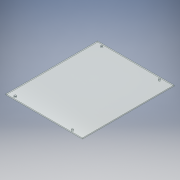
# Autodesk Inventor part: Perspex base
Saved by Autodesk Inventor 2019 (Build 230136000, 136)
## iProperties
Created: 2021-03-22
Part Number: Perspex base
Material: Glass
Document SubType Name: Modeling
Designer: User
Density: 2.18 g/cm^3
Appearance: Clear
Author: User
Autodesk Inventor part; units mm, degrees
ref_plane "YZ Plane" through (0, 0, 0) normal (1, 0, 0) x (0, 1, 0)
ref_plane "XZ Plane" through (0, 0, 0) normal (0, 1, 0) x (-1, 0, 0)
ref_plane "XY Plane" through (0, 0, 0) normal (0, 0, 1) x (1, 0, 0)
sketch "Sketch1" plane through (0, 0, 0) normal (0, 1, 0) x (-1, 0, 0)
  line L0 (300, 0) -> (-11, 0)
  line L1 (-11, 0) -> (-11, -373)
  line L2 (-11, -373) -> (300, -373)
  line L3 (300, -373) -> (300, 0)
  point P0 (0, 0)
  dimension "d0" = 373
  dimension "d1" = 311
  dimension "d2" = 300
  dimension "d3" = 0
  constraints: 8 end point, 2 parallel, 1 horizontal, 1 perpendicular
  measures "d0" distance between parallel lines of L2 L0
  measures "d1" distance between parallel lines of L3 L1
  measures "d2" distance from line of point (0, 0) L3
  measures "d3" distance from line of point (0, 0) L0
extrude "Extrusion1" add sketch "Sketch1" along normal mid plane 4
sketch "Sketch2" plane through (0, 2, 0) normal (0, 1, 0) x (1, 0, 0)
  circle A0 centre (-39, 9.5) radius 4
  circle A1 centre (-39, 363.5) radius 4
  circle A2 centre (-274, 12) radius 4.75
  circle A3 centre (-274, 363.5) radius 4
  line L0 (11, 373) -> (-300, 373) projected
  line L1 (-300, 373) -> (-300, 0) projected
  line L2 (-300, 0) -> (11, 0) projected
  line L3 (11, 0) -> (11, 373) projected
  point P0 (0, 0)
  dimension "d6" = 8
  dimension "d7" = 8
  dimension "d8" = 9.5
  dimension "d9" = 8
  dimension "d10" = 9.5
  dimension "d13" = 12
  dimension "d14" = 9.5
  dimension "d15" = 50
  dimension "d16" = 50
  dimension "d17" = 9.5
  dimension "d20" = 235
  dimension "d21" = 235
  constraints: 4 centre point
  measures "d6" diameter of A0
  measures "d7" diameter of A1
  measures "d8" diameter of A2
  measures "d9" diameter of A3
  measures "d10" distance from line of L0 A3.centre
  measures "d13" distance from line of L2 A2.centre
  measures "d14" distance from line of A0.centre L2
  measures "d15" distance from line of L3 A0.centre
  measures "d16" distance from line of L3 A1.centre
  measures "d17" distance from line of L0 A1.centre
  measures "d20" horizontal distance of A2.centre A0.centre
  measures "d21" distance of A3.centre A1.centre
extrude "Extrusion2" cut sketch "Sketch2" against normal blind 4 contours A0 | A1 | A2 | A3
body "Solid1"
